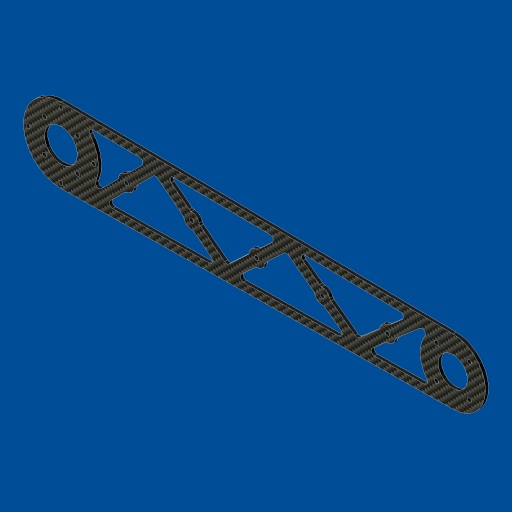
# Autodesk Inventor part: LowerArmPlate
Saved by Autodesk Inventor 2023 (Build 270158030, 158C)
## iProperties
Created: 2023-03-01
Part Number: LowerArmPlate
Material: CFRP
Document SubType Name: Modeling
Designer: kumpu
Density: 1.43 g/cm^3
Appearance: Glossy - Black
Author: kumpu
Autodesk Inventor part; units mm, degrees
ref_plane "YZ Plane" through (0, 0, 0) normal (1, 0, 0) x (0, 1, 0)
ref_plane "XZ Plane" through (0, 0, 0) normal (0, 1, 0) x (-1, 0, 0)
ref_plane "XY Plane" through (0, 0, 0) normal (0, 0, 1) x (1, 0, 0)
sketch "Sketch1" plane through (0, 0, 0) normal (0, 0, 1) x (1, 0, 0)
  line L0 (0, 0) -> (381, 0) construction
  line L1 (0.4564, -36.5096) -> (381.3969, -31.7475)
  line L2 (381.3969, 31.7475) -> (0.4564, 36.5096)
  arc A0 (0.4564, 36.5096) -> (0.4564, -36.5096) centre (0, 0) ccw
  arc A1 (381.3969, -31.7475) -> (381.3969, 31.7475) centre (381, 0) ccw
  circle A2 centre (0, 0) radius 16
  circle A3 centre (381, 0) radius 14.2875
  point P0 (190.5, 0)
  dimension "d0" = 381
  dimension "d2" = 32
  dimension "d5" = 36.5125
  dimension "d6" = 31.75
  dimension "d7" = 28.575
  constraints: 8 end point, 4 centre point, 4 point on circle, 4 tangent, 2 coincident, 1 horizontal, 1 midpoint
  measures "d0" distance of L0.start L0.end
  measures "d2" diameter of A2
  measures "d5" radius of A0
  measures "d6" radius of A1
  measures "d7" diameter of A3
extrude "Extrusion1" add sketch "Sketch1" along normal mid plane 3
sketch "Sketch2" plane through (0, 0, -1.5) normal (0, 0, -1) x (-1, 0, 0)
  circle A0 centre (0, -32) radius 2
  circle A1 centre (-16, -16) radius 2
  line L0 (0, -32) -> (0, 0) construction
  line L1 (0, 0) -> (-16, -16) construction
  line L2 (0, 0) -> (-63.5, 0) construction
  circle A2 centre (-63.5, 0) radius 2
  circle A3 centre (32, 0) radius 2
  circle A4 centre (16, -16) radius 2
  circle A5 centre (0, 32) radius 2
  circle A6 centre (16, 16) radius 2
  circle A7 centre (-32, 0) radius 2
  circle A8 centre (-16, 16) radius 2
  circle A9 centre (-127, 0) radius 2
  circle A10 centre (-190.5, 0) radius 2
  circle A11 centre (-254, 0) radius 2
  circle A12 centre (-317.5, 0) radius 2
  line L3 (-22.684, 28.6112) -> (-84.1585, 27.8427)
  line L4 (-84.1585, 27.8427) -> (-63.924, 7.6082)
  line L5 (-71.1082, 0.424) -> (-91.6778, 20.9935)
  line L6 (-91.6778, 20.9935) -> (-119.3984, -0.5294)
  line L7 (-345.9608, 24.5699) -> (-91.254, 27.754) construction
  line L8 (-0.4564, 36.5096) -> (-381.3969, 31.7475) construction
  line L9 (-35.0433, -28.4567) -> (-91.254, 27.754) construction
  line L10 (-91.254, 27.754) -> (-161.6132, -26.8744) construction
  line L11 (-161.6132, -26.8744) -> (-218.6208, 26.1618) construction
  line L12 (-218.6208, 26.1618) -> (-288.2029, -25.2919) construction
  line L13 (-288.2029, -25.2919) -> (-345.9608, 24.5699) construction
  line L14 (-35.0433, -28.4567) -> (-288.2029, -25.2919) construction
  line L15 (-381.3969, -31.7475) -> (-0.4564, -36.5096) construction
  circle A13 centre (-397, -16) radius 2
  line L16 (-397, -16) -> (-381, 0) construction
  circle A14 centre (-381, 0) radius 14.2875 construction
  circle A15 centre (-365, -16) radius 2
  circle A16 centre (-365, 16) radius 2
  circle A17 centre (-397, 16) radius 2
  line L17 (-316.5204, -7.5568) -> (-296.091, -25.1933)
  line L18 (-296.091, -25.1933) -> (-360.6682, -24.3861)
  arc A18 (-360.6682, -24.3861) -> (-353.879, 16.5079) centre (-381, 0) ccw
  arc A19 (-325.1188, -0.1339) -> (-316.5204, -7.5568) centre (-317.5, 0) ccw
  arc A20 (-309.8812, 0.1339) -> (-318.4796, 7.5568) centre (-317.5, 0) ccw
  arc A21 (-252.4537, 7.4615) -> (-261.5871, 0.7076) centre (-254, 0) ccw
  arc A22 (-255.5463, -7.4615) -> (-246.4129, -0.7076) centre (-254, 0) ccw
  arc A23 (-198.1185, 0.1493) -> (-189.8019, -7.588) centre (-190.5, 0) ccw
  arc A24 (-182.8815, -0.1493) -> (-191.1981, 7.588) centre (-190.5, 0) ccw
  arc A25 (-125.6293, 7.4957) -> (-134.6016, 0.5294) centre (-127, 0) ccw
  arc A26 (-128.3707, -7.4957) -> (-119.3984, -0.5294) centre (-127, 0) ccw
  arc A27 (-71.1082, 0.424) -> (-63.076, -7.6082) centre (-63.5, 0) ccw
  arc A28 (-55.8918, -0.424) -> (-63.924, 7.6082) centre (-63.5, 0) ccw
  circle A29 centre (-63.5, 0) radius 5.08 construction
  circle A30 centre (-127, 0) radius 5.08 construction
  circle A31 centre (-190.5, 0) radius 5.08 construction
  circle A32 centre (-254, 0) radius 5.08 construction
  circle A33 centre (-317.5, 0) radius 5.08 construction
  line L19 (-318.4796, 7.5568) -> (-338.2978, 24.6657)
  line L20 (-338.2978, 24.6657) -> (-227.3118, 26.0531)
  line L21 (-227.3118, 26.0531) -> (-252.4537, 7.4615)
  line L22 (-261.5871, 0.7076) -> (-287.9576, -18.7925)
  line L23 (-287.9576, -18.7925) -> (-309.8812, 0.1339)
  line L24 (-189.8019, -7.588) -> (-169.1728, -26.7799)
  line L25 (-169.1728, -26.7799) -> (-279.8009, -25.397)
  line L26 (-279.8009, -25.397) -> (-255.5463, -7.4615)
  line L27 (-198.1185, 0.1493) -> (-218.9924, 19.569)
  line L28 (-218.9924, 19.569) -> (-246.4129, -0.7076)
  line L29 (-182.8815, -0.1493) -> (-161.3161, -20.2123)
  line L30 (-161.3161, -20.2123) -> (-134.6016, 0.5294)
  line L31 (-125.6293, 7.4957) -> (-99.673, 27.6487)
  line L32 (-99.673, 27.6487) -> (-211.2617, 26.2538)
  line L33 (-211.2617, 26.2538) -> (-191.1981, 7.588)
  line L34 (-63.076, -7.6082) -> (-42.3185, -28.3657)
  line L35 (-42.3185, -28.3657) -> (-153.461, -26.9763)
  line L36 (-153.461, -26.9763) -> (-128.3707, -7.4957)
  line L37 (-38.9317, -17.3841) -> (-55.8918, -0.424)
  arc A34 (-0.4564, -36.5096) -> (-0.4564, 36.5096) centre (0, 0) ccw construction
  arc A35 (-381.3969, 31.7475) -> (-381.3969, -31.7475) centre (-381, 0) ccw construction
  line L38 (-325.1188, -0.1339) -> (-349.0921, 20.562)
  arc A36 (-22.684, 28.6112) -> (-33.7517, -13.9279) centre (0, 0) ccw
  arc A37 (-38.9317, -17.3841) -> (-33.7517, -13.9279) centre (-36.6866, -15.1391) ccw
  arc A38 (-349.0921, 20.562) -> (-353.879, 16.5079) centre (-351.1669, 18.1587) ccw
  dimension "d8" = 45
  dimension "d9" = 16
  dimension "d10" = 32
  dimension "d11" = 4
  dimension "d14" = 360
  dimension "d16" = 63.5
  dimension "d17" = 4
  dimension "d20" = 63.5
  dimension "d25" = 7.62
  dimension "d26" = 7.62
  dimension "d27" = 45
  dimension "d28" = 45
  dimension "d29" = 16
  dimension "d32" = 360
  dimension "d34" = 10.16
  dimension "d35" = 7.62
  dimension "d36" = 3.175
  constraints: 74 end point, 36 centre point, 28 point on circle, 21 collinear, 21 parallel, 18 equal radius, 14 tangent, 13 concentric, 9 coincident, 8 point on line, 2 horizontal, 1 vertical, 34 other
  measures "d8" angle of L0 L1
  measures "d9" distance from line of L2 L1.end
  measures "d10" distance of L0.start L0.end
  measures "d11" diameter of A0
  measures "d16" distance of L2.end L0.end
  measures "d17" diameter of A2
  measures "d20" distance of A2.centre A9.centre
  measures "d25" distance between parallel lines of L14 L15
  measures "d26" distance between parallel lines of L8 L7
  measures "d27" angle of L2 L9
  measures "d28" angle of L2 L16
  measures "d29" horizontal distance of L16.end L16.start
  measures "d34" diameter of A33
  measures "d35" radius of A22
  measures "d36" radius of A37
extrude "Extrusion2" cut sketch "Sketch2" against normal through all
fillet "Fillet1" radius 3.175 36 edges at (22.684, 28.6112, 0) (42.3185, -28.3657, 0) (84.1585, 27.8427, 0) (91.6778, 20.9935, 0) (99.673, 27.6487, 0) (55.8918, -0.424, 0) (63.924, 7.6082, 0) (71.1082, 0.424, 0) (63.076, -7.6082, 0) (128.3707, -7.4957, 0) (119.3984, -0.5294, 0) (125.6293, 7.4957, 0) (134.6016, 0.5294, 0) (153.461, -26.9763, 0) (161.3161, -20.2123, 0) (169.1728, -26.7799, 0) (182.8815, -0.1493, 0) (189.8019, -7.588, 0) (198.1185, 0.1493, 0) (191.1981, 7.588, 0) (211.2617, 26.2538, 0) (218.9924, 19.569, 0) (227.3118, 26.0531, 0) (246.4129, -0.7076, 0) (252.4537, 7.4615, 0) (261.5871, 0.7076, 0) (255.5463, -7.4615, 0) (279.8009, -25.397, 0) (287.9576, -18.7925, 0) (296.091, -25.1933, 0) (309.8812, 0.1339, 0) (318.4796, 7.5568, 0) (325.1188, -0.1339, 0) (316.5204, -7.5568, 0) (338.2978, 24.6657, 0) (360.6682, -24.3861, 0)
equation "\"d20\" = d16"
equation "\"d26\" = d25"
body "Solid1"
